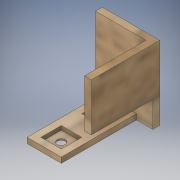
# Autodesk Inventor part: Slider
Saved by Autodesk Inventor 2017 (Build 210142000, 142)
## iProperties
Created: 2017-05-30
Part Number: Slider
Material: Wood (Maple)
Document SubType Name: Modeling
Designer: sensor
Density: 0.67 g/cm^3
Appearance: Natural Maple - Glossy Dark Tint
Author: sensor
Autodesk Inventor part; units mm, degrees
ref_plane "YZ Plane" through (0, 0, 0) normal (1, 0, 0) x (0, 1, 0)
ref_plane "XZ Plane" through (0, 0, 0) normal (0, 1, 0) x (-1, 0, 0)
ref_plane "XY Plane" through (0, 0, 0) normal (0, 0, 1) x (1, 0, 0)
sketch "BackwithHoles" plane through (0, 0, 0) normal (0, 1, 0) x (-1, 0, 0)
  line L0 (0, 0) -> (25, 0)
  line L1 (25, 0) -> (25, 60)
  line L2 (25, 60) -> (0, 60)
  line L3 (0, 60) -> (0, 0)
  circle A0 centre (12.5, 47.5) radius 3
  circle A1 centre (12.5, 17.5) radius 3
  dimension "d8" = 25
  dimension "d9" = 60
  dimension "d10" = 6
  dimension "d11" = 6
  dimension "d12" = 12.5
  dimension "d13" = 12.5
  dimension "d14" = 12.5
  dimension "d15" = 17.5
  constraints: 8 end point, 2 centre point, 2 parallel, 1 horizontal, 1 perpendicular
  measures "d8" distance of L1.end L2.end
  measures "d9" distance of L0.end L1.end
  measures "d10" diameter of A0
  measures "d11" diameter of A1
  measures "d12" distance from line of L3 A0.centre
  measures "d13" distance from line of A1.centre L3
  measures "d14" distance from line of A0.centre L2
  measures "d15" distance from line of L0 A1.centre
extrude "Extrusion1" add sketch "BackwithHoles" along normal blind 4
sketch "Bottom" plane through (0, 4, 0) normal (0, 1, 0) x (1, 0, 0)
  line L0 (0, -60) -> (0, 0) projected
  line L1 (0, 0) -> (-25, 0) projected
  line L2 (0, -5) -> (-25, -5)
  line L3 (-25, -5) -> (-25, 0)
  line L4 (-25, 0) -> (0, 0)
  line L5 (0, 0) -> (0, -5)
  dimension "d18" = 5
  constraints: 8 end point, 2 parallel, 1 horizontal, 1 perpendicular, 1 point on line
  measures "d18" distance of L0.end L2.start
extrude "Extrusion2" add sketch "Bottom" along normal blind 15
sketch "HolesonBottom" plane through (-25, 4, 5) normal (0, 0, 1) x (1, 0, 0)
  circle A0 centre (17.5, 7.5) radius 2.5
  circle A1 centre (5, 7.5) radius 2.5
  line L0 (25, 0) -> (25, 15) projected
  line L1 (0, 0) -> (0, 15) projected
  line L2 (0, 0) -> (25, 0) projected
  point P0 (25, -4)
  dimension "d21" = 5
  dimension "d22" = 5
  dimension "d23" = 7.5
  dimension "d24" = 5
  dimension "d25" = 7.5
  dimension "d26" = 7.5
  dimension "d27" = 12.5
  constraints: 2 centre point
  measures "d21" diameter of A0
  measures "d22" diameter of A1
  measures "d23" distance from line of L0 A0.centre
  measures "d24" distance from line of L1 A1.centre
  measures "d25" distance from line of L2 A0.centre
  measures "d26" distance from line of L2 A1.centre
  measures "d27" distance of A1.centre A0.centre
hole "Hole1" at (-7.5, 11.5, 5) at (-20, 11.5, 5) direction (0, 0, -1) diameter 5.86 end through all
sketch "TopSquare" plane through (0, 4, 0) normal (0, 1, 0) x (1, 0, 0)
  line L0 (-20, -55) -> (-5, -55)
  line L1 (-5, -55) -> (-5, -40)
  line L2 (-5, -40) -> (-20, -40)
  line L3 (-20, -40) -> (-20, -55)
  line L4 (-25, -60) -> (0, -60) projected
  line L5 (0, -60) -> (0, -5) projected
  point P0 (0, 0)
  dimension "d35" = 5
  dimension "d36" = 15
  dimension "d37" = 15
  dimension "d38" = 5
  constraints: 8 end point, 2 parallel, 1 horizontal, 1 perpendicular
  measures "d35" distance between parallel lines of L4 L0
  measures "d36" distance of L1.end L2.end
  measures "d37" distance of L2.end L0.start
  measures "d38" distance between parallel lines of L5 L1
extrude "Extrusion3" cut sketch "TopSquare" against normal blind 3
sketch "BottomSquare" plane through (0, 4, 0) normal (0, 1, 0) x (1, 0, 0)
  line L0 (-20, -25) -> (-5, -25)
  line L1 (-5, -25) -> (-5, -10)
  line L2 (-5, -10) -> (-20, -10)
  line L3 (-20, -10) -> (-20, -25)
  line L4 (0, -60) -> (0, -5) projected
  line L5 (-20, -40) -> (-5, -40) projected
  point P0 (0, 0)
  point P1 (-20, -40)
  dimension "d41" = 15
  dimension "d42" = 15
  dimension "d43" = 5
  dimension "d44" = 30
  constraints: 8 end point, 2 parallel, 1 horizontal, 1 perpendicular
  measures "d41" distance of L2.end L0.start
  measures "d42" distance of L0.start L0.end
  measures "d43" distance between parallel lines of L4 L1
  measures "d44" distance between parallel lines of L2 L5
extrude "Extrusion4" cut sketch "BottomSquare" against normal blind 3
sketch "BottomExtrusion" plane through (0, 19, 0) normal (0, 1, 0) x (1, 0, 0)
  line L0 (0, 0) -> (-25, 0) projected
  line L1 (-25, 0) -> (-25, -5) projected
  line L2 (0, 0) -> (-25, 0)
  line L3 (-25, 0) -> (-25, -5)
  line L4 (-25, -5) -> (0, -5)
  line L5 (0, -5) -> (0, 0)
  constraints: 8 end point, 2 parallel, 1 horizontal, 1 perpendicular
extrude "Extrusion7" add sketch "BottomExtrusion" along normal blind 23
sketch "BottomExteriorExtrusion" plane through (0, 0, 60) normal (1, 0, 0) x (0, 0, -1)
  line L0 (55, 42) -> (60, 42) projected
  line L1 (60, 0) -> (55, 0)
  line L2 (55, 0) -> (55, 42)
  line L3 (55, 42) -> (60, 42)
  line L4 (60, 42) -> (60, 0)
  constraints: 8 end point, 2 parallel, 1 horizontal, 1 perpendicular
extrude "Extrusion8" add sketch "BottomExteriorExtrusion" along normal blind 12
sketch "ContainingWall" plane through (-25, 4, 5) normal (0, 0, 1) x (1, 0, 0)
  line L0 (37, -4) -> (37, 38) projected
  line L1 (0, 38) -> (37, 38) projected
  line L2 (37, 15) -> (32, 15)
  line L3 (32, 15) -> (32, 38)
  line L4 (32, 38) -> (37, 38)
  line L5 (37, 38) -> (37, 15)
  point P0 (25, -4)
  dimension "d56" = 5
  dimension "d57" = 23
  constraints: 8 end point, 2 parallel, 2 point on line, 1 horizontal, 1 perpendicular
  measures "d56" distance of L2.start L2.end
  measures "d57" distance of L2.end L3.end
extrude "Extrusion9" add sketch "ContainingWall" along normal blind 45
sketch "ContainingWallExtension" plane through (0, 42, 0) normal (0, 1, 0) x (1, 0, 0)
  line L0 (12, 0) -> (12, -50) projected
  line L1 (7, -50) -> (12, -50) projected
  line L2 (12, -50) -> (7, -50)
  line L3 (-25, -5) -> (7, -5) projected
  line L4 (7, -50) -> (7, -5)
  line L5 (7, -5) -> (-25, -5)
  line L6 (-25, 0) -> (12, 0) projected
  line L7 (-25, -5) -> (-25, 0)
  line L8 (-25, 0) -> (12, 0)
  line L9 (12, 0) -> (12, -50)
  point P0 (0, 0)
  constraints: 12 end point, 3 collinear, 3 perpendicular
extrude "Extrusion10" add sketch "ContainingWallExtension" along normal blind 12
sketch "AnteriorBottomExtension" plane through (-25, 0, 0) normal (-1, 0, 0) x (0, 0, 1)
  line L0 (5, 0) -> (0, 0) projected
  line L1 (0, 0) -> (0, 54) projected
  line L2 (0, 0) -> (0, 54)
  line L3 (5, 19) -> (5, 54) projected
  line L4 (0, 54) -> (5, 54)
  line L5 (5, 19) -> (5, 0) projected
  line L6 (5, 54) -> (5, 0)
  line L7 (5, 0) -> (0, 0)
  constraints: 8 end point, 3 perpendicular, 1 vertical
extrude "Extrusion11" add sketch "AnteriorBottomExtension" along normal blind 5
body "Solid1"
